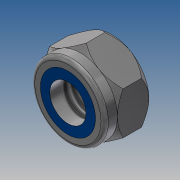
# Autodesk Inventor part: M6 nyloc
Saved by Autodesk Inventor 2014 (Build 180170000, 170)
## iProperties
Created: 2013-10-03
Part Number: M6 nyloc
Material: Steel, Carbon
Document SubType Name: Modeling
Designer: Andrew
Mass: 3.02006 g
Surface Area: 4.06519 cm^2
Volume: 0.383743 cm^3
Density: 7.87 g/cm^3
Appearance: Semi-Polished
Author: Andrew
Autodesk Inventor part; units mm, degrees
ref_plane "YZ Plane" through (0, 0, 0) normal (1, 0, 0) x (0, 1, 0)
ref_plane "XZ Plane" through (0, 0, 0) normal (0, 1, 0) x (-1, 0, 0)
ref_plane "XY Plane" through (0, 0, 0) normal (0, 0, 1) x (1, 0, 0)
sketch "Sketch1" plane through (0, 0, 0) normal (0, 1, 0) x (-1, 0, 0)
  line L0 (5, 2.8868) -> (5, -2.8868)
  line L1 (5, -2.8868) -> (0, -5.7735)
  line L2 (0, -5.7735) -> (-5, -2.8868)
  line L3 (-5, -2.8868) -> (-5, 2.8868)
  line L4 (-5, 2.8868) -> (0, 5.7735)
  line L5 (0, 5.7735) -> (5, 2.8868)
  point P0 (0, 0)
  point P1 (0, 0)
  dimension "d0" = 10
  constraints: 12 end point, 1 coincident, 1 vertical, 13 other
  measures "d0" distance between parallel lines of L0 L3
extrude "Extrusion1" add sketch "Sketch1" along normal blind 6
sketch "Sketch2" plane through (0, 6, 0) normal (0, 1, 0) x (1, 0, 0)
  point P0 (0, 0)
  point P1 (0, 0)
  constraints: 1 coincident
hole "Hole1" at (0, 6, 0) direction (0, -1, 0) diameter 4.917 end through all thread size "M6x1" class "6H" standard "ISO Metric profile"
sketch "Sketch3" plane through (0, 0, 0) normal (1, 0, 0) x (0, 1, 0)
  line L0 (0, 0) -> (9.121, 0)
  line L1 (0, 5.7735) -> (6, 5.7735) projected
  line L2 (2.5, 5.7735) -> (1.7265, 5)
  line L3 (1.7265, 5) -> (0, 5)
  line L4 (0, 5) -> (0, 5.7735)
  line L5 (6, 5.7735) -> (6, 2.8868) projected
  dimension "d10" = 10
  dimension "d11" = 3.5
  dimension "d12" = 45
  constraints: 8 end point, 1 horizontal, 1 parallel, 1 perpendicular, 1 point on line
  measures "d10" diameter of L3 L0
  measures "d11" distance from line of L5 L2.start
  measures "d12" angle of L1 L2
revolve "Revolution1" cut sketch "Sketch3" angle 360 about axis through (0, 0, 0) along (0, 1, 0)
fillet "Fillet1" radius 0.5 1 edges at (0, 0, -5)
sketch "Sketch4" plane through (0, 0, 0) normal (0, -1, 0) x (1, 0, 0)
  circle A0 centre (0, 0) radius 4.5 projected
  circle A1 centre (0, 0) radius 3.75
  dimension "d15" = 7.5
  constraints: 1 centre point, 1 coincident
  measures "d15" diameter of A1
split_face "Split1"
sketch "Sketch5" plane through (0, 0, 0) normal (1, 0, 0) x (0, 1, 0)
  line L0 (0, 0) -> (10.6904, 0)
  line L1 (2.5, 5.7735) -> (6, 5.7735) projected
  line L2 (5, 5.7735) -> (6, 5)
  line L3 (6, 5) -> (6, 5.7735)
  line L4 (6, 5) -> (10.4328, 5)
  dimension "d16" = 1
  dimension "d17" = 10
  constraints: 8 end point, 2 perpendicular, 1 horizontal, 1 point on line
  measures "d16" distance from line of L3 L2.start
  measures "d17" diameter of L4 L0
revolve "Revolution2" cut sketch "Sketch5" angle 360 about axis through (0, 0, 0) along (0, 1, 0)
chamfer "Chamfer1" distance 0.5 angle 45 1 edges at (0, 6, -2.4585)
body "Solid1"
